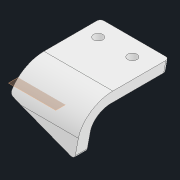
# Autodesk Inventor part: scara-base28
Saved by Autodesk Inventor 2022 (Build 260153000, 153)
## iProperties
Created: 2021-11-05
Part Number: scara-base28
Material: ABS プラスチック
Document SubType Name: Modeling
Designer: Yuta Kage
Density: 1.06 g/cm^3
Appearance: 滑らか - 白
Author: Yuta Kage
Autodesk Inventor part; units mm, degrees
ref_plane "YZ Plane" through (0, 0, 0) normal (1, 0, 0) x (0, 1, 0)
ref_plane "XZ Plane" through (0, 0, 0) normal (0, 1, 0) x (-1, 0, 0)
ref_plane "XY Plane" through (0, 0, 0) normal (0, 0, 1) x (1, 0, 0)
sketch "スケッチ1" plane through (0, 0, 0) normal (0, 0, 1) x (1, 0, 0)
  line L0 (0, 0) -> (410.7754, -157.6819) construction
  line L1 (0, 0) -> (440, 0) construction
  line L2 (460, -20) -> (-20, -20)
  line L3 (-20, -20) -> (-20, 20) construction
  line L4 (-20, 20) -> (460, 20) construction
  line L5 (460, 20) -> (460, -20) construction
  line L6 (460, -20) -> (-20, 20) construction
  line L7 (-20, -20) -> (460, 20) construction
  line L8 (-25.839, -11.5042) -> (422.2796, -183.5209) construction
  line L9 (422.2796, -183.5209) -> (436.6144, -146.1776) construction
  line L10 (436.6144, -146.1776) -> (-11.5042, 25.839)
  line L11 (-11.5042, 25.839) -> (-25.839, -11.5042) construction
  line L12 (-25.839, -11.5042) -> (436.6144, -146.1776) construction
  line L13 (422.2796, -183.5209) -> (-11.5042, 25.839) construction
  circle A0 centre (0, 0) radius 150
  circle A1 centre (0, 0) radius 190
  line L14 (148.6607, -20) -> (145.9541, -34.6036)
  line L15 (188.9444, -20) -> (183.5622, -49.04)
  point P0 (220, 0)
  point P1 (205.3877, -78.8409)
  dimension "d0" = 159
  dimension "d1" = 440
  dimension "d2" = 440
  dimension "d3" = 40
  dimension "d4" = 480
  dimension "d5" = 480
  dimension "d6" = 40
  dimension "d7" = 20
  dimension "d8" = 300
  dimension "d30" = 40
  constraints: 32 end point, 6 midpoint, 5 parallel, 4 point on circle, 4 point on line, 2 centre point, 2 coincident, 2 horizontal, 2 perpendicular
  measures "d0" angle of L1 L0
  measures "d1" distance of L0.start L0.end
  measures "d2" distance of L0.start L1.end
  measures "d3" distance of L2.end L3.end
  measures "d4" distance of L3.end L4.end
  measures "d5" distance of L9.end L10.end
  measures "d6" distance between parallel lines of L8 L10
  measures "d7" distance from line of L11 L0.start
  measures "d8" diameter of A0
  measures "d30" radial gap between concentric circles of A1 A0
extrude "押し出し1" add sketch "スケッチ1" along normal mid plane 50 contours L15 L10 A0 L2 | A0 L14
ref_plane "作業平面1" through (148.6607, -27, 25) normal (0, 1, 0) x (1, 0, 0)
sketch "スケッチ2" plane through (148.6607, -27, 25) normal (0, 1, 0) x (1, 0, 0)
  line L0 (-2.7066, 7) -> (40.2837, 7)
  line L1 (40.2837, 7) -> (40.2837, 50)
  line L2 (40.2837, 50) -> (-2.7066, 50)
  line L3 (-2.7066, 50) -> (-2.7066, 7)
  point P0 (-148.6607, 25)
  constraints: 8 end point, 2 parallel, 1 horizontal, 1 perpendicular
extrude "押し出し2" cut sketch "スケッチ2" against normal blind 50
fillet "フィレット1" radius 10 1 edges at (167.5052, -27, 18)
fillet "フィレット2" radius 17 1 edges at (168.8026, -20, 25)
fillet "フィレット3" radius 2 4 edges at (183.5622, -49.04, 21.5) (145.9541, -34.6036, 21.2694) (188.2957, -23.5, -25) (148.012, -23.5, -25)
sketch "スケッチ3" plane through (148.6607, -27, 25) normal (0, -1, 0) x (1, 0, 0)
  line L0 (38.9864, -50) -> (-1.2974, -50) projected
  line L1 (-1.2974, -48) -> (-1.2974, -17) projected
  point P0 (-148.6607, -25)
  point P1 (8.7026, -40)
  point P2 (37.3904, -50)
  point P3 (50.415, -50)
  point P4 (28.7026, -40)
  dimension "d20" = 10
  dimension "d29" = 20
  dimension "d31" = 10
  constraints: 1 horizontal alignment
  measures "d20" distance from line of L0 point (8.703, -40)
  measures "d29" distance of point (8.703, -40) point (28.703, -40)
  measures "d31" distance from line of L1 point (8.703, -40)
hole "穴1" at (157.3633, -27, -15) at (177.3633, -27, -15) direction (0, 1, 0) diameter 5.5 end through all clearance for "Flat Head Machine Screw" size "M5" standard "Ansi Metric M Profile"
